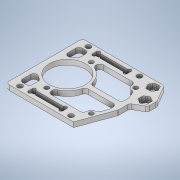
# Autodesk Inventor part: Trunk_vertical_frame_04
Saved by Autodesk Inventor 2020.4 (Build 244396000, 396)
## iProperties
Created: 2021-09-10
Part Number: Trunk_vertical_frame_04
Material: アルミニウム 2014-T4
Document SubType Name: Modeling
Designer: Masato Kubotera
Density: 2.8 g/cm^3
Appearance: 滑らか - 淡い灰色
Mass: 10.7602 g
Surface Area: 49.1447 cm^2
Volume: 3.84295 cm^3
Author: Masato Kubotera
Autodesk Inventor part; units mm, degrees
ref_plane "YZ Plane" through (0, 0, 0) normal (1, 0, 0) x (0, 1, 0)
ref_plane "XZ Plane" through (0, 0, 0) normal (0, 1, 0) x (-1, 0, 0)
ref_plane "XY Plane" through (0, 0, 0) normal (0, 0, 1) x (1, 0, 0)
derived "Trunk_vertical_frame_03.ipt"
sketch "スケッチ1" plane through (0, 0, 0) normal (0, 0, 1) x (1, 0, 0)
  circle A0 centre (0, 0) radius 11
  line L0 (1, 13.5) -> (28, 13.5) construction
  line L1 (28, 13.5) -> (28, -13.5) construction
  line L2 (28, -13.5) -> (1, -13.5) construction
  line L3 (1, -13.5) -> (1, 13.5) construction
  line L4 (1, 13.5) -> (28, -13.5) construction
  line L5 (28, 13.5) -> (1, -13.5) construction
  line L6 (-12, 16) -> (39.5, 16) construction
  line L7 (39.5, 16) -> (39.5, -16) construction
  line L8 (39.5, -16) -> (-12, -16) construction
  line L9 (-12, -16) -> (-12, 16) construction
  line L10 (-12, 16) -> (39.5, -16) construction
  line L11 (39.5, 16) -> (-12, -16) construction
  circle A1 centre (1, 13.5) radius 1.35
  arc A2 (0, 16) -> (-12, 10.583) centre (0, 0) ccw construction
  line L12 (-12, 0) -> (39.5, 0) construction
  circle A3 centre (28, 13.5) radius 1.35
  arc A4 (-12, -10.583) -> (0, -16) centre (0, 0) ccw construction
  circle A5 centre (28, -13.5) radius 1.35
  circle A6 centre (1, -13.5) radius 1.35
  arc A7 (0, 16.01) -> (-12.01, 10.5868) centre (0, 0) ccw construction
  line L13 (0, 16.01) -> (39.51, 16.01) construction
  line L14 (39.51, 16.01) -> (39.51, 13.26) construction
  line L15 (-12.01, 10.5868) -> (-12.01, 0) construction
  arc A8 (-11.4729, 11.1666) -> (-12.01, 9.8444) centre (-11.0278, 10.2156) ccw construction
  line L16 (-12.01, 10.5868) -> (-11.0278, 10.2156) construction
  arc A9 (39.51, 14.5251) -> (38.0251, 16.01) centre (38.7675, 15.2675) ccw construction
  line L17 (38.7675, 15.2675) -> (39.51, 16.01) construction
  arc A10 (38.0251, -16.01) -> (39.51, -14.5251) centre (38.7675, -15.2675) ccw construction
  line L18 (-12.01, -10.5868) -> (-12.01, 0) construction
  arc A11 (-12.01, -9.8444) -> (-11.4729, -11.1666) centre (-11.0278, -10.2156) ccw construction
  arc A12 (-12.01, -10.5868) -> (0, -16.01) centre (0, 0) ccw construction
  line L19 (0, -16.01) -> (39.51, -16.01) construction
  line L20 (39.51, 13.26) -> (42.01, 13.26) construction
  line L21 (42.01, 13.26) -> (42.01, -1.76) construction
  line L22 (42.01, -1.76) -> (39.51, -1.76) construction
  line L23 (39.51, -1.76) -> (39.51, -14.5251) construction
  line L24 (39.5, 13.25) -> (42, 13.25) construction
  line L25 (42, 13.25) -> (42, -1.75) construction
  line L26 (42, -1.75) -> (39.5, -1.75) construction
  line L27 (42, 5.75) -> (39.5, 5.75) construction
  arc A13 (42.01, 11.7751) -> (40.5251, 13.26) centre (41.2675, 12.5175) ccw construction
  line L28 (41.2675, 12.5175) -> (42.01, 13.26) construction
  arc A14 (40.5251, -1.76) -> (42.01, -0.2751) centre (41.2675, -1.0175) ccw construction
  circle A15 centre (-15.5, 19) radius 1.55 construction
  line L29 (-18, 22) -> (-13, 22) construction
  line L30 (-13, 22) -> (-13, -10.5) construction
  line L31 (-13, -10.5) -> (-18, -10.5) construction
  line L32 (-18, -10.5) -> (-18, 22) construction
  line L33 (-18, 22) -> (-13, -10.5) construction
  line L34 (-13, 22) -> (-18, -10.5) construction
  line L35 (-18, 5.75) -> (-13, 5.75) construction
  line L36 (-15.5, 22) -> (-15.5, -10.5) construction
  line L37 (-18, 13.25) -> (-15.5, 13.25) construction
  line L38 (-15.5, 13.25) -> (-15.5, -1.75) construction
  line L39 (-15.5, -1.75) -> (-18, -1.75) construction
  line L40 (-18, 13.25) -> (-15.5, -1.75) construction
  line L41 (-15.5, 13.25) -> (-18, -1.75) construction
  line L42 (-15.49, -1.76) -> (-18.01, -1.76) construction
  line L43 (-18.01, -1.76) -> (-18.01, 13.26) construction
  line L44 (-18.01, 13.26) -> (-15.49, 13.26) construction
  line L45 (-15.49, 13.26) -> (-15.49, -1.76) construction
  line L46 (-15.49, -1.76) -> (-18.01, 13.26) construction
  line L47 (-18.01, -1.76) -> (-15.49, 13.26) construction
  line L48 (-16.75, 13.26) -> (-16.75, -1.76) construction
  arc A16 (-18.01, 13.26) -> (-18.01, 11.16) centre (-18.01, 12.21) ccw construction
  arc A17 (-15.49, 11.16) -> (-15.49, 13.26) centre (-15.49, 12.21) ccw construction
  arc A18 (-18.01, 0.34) -> (-18.01, -1.76) centre (-18.01, -0.71) ccw construction
  arc A19 (-15.49, -1.76) -> (-15.49, 0.34) centre (-15.49, -0.71) ccw construction
  circle A20 centre (-15.5, -7.5) radius 1.55 construction
  line L49 (14.5, 16) -> (14.5, -16) construction
  circle A21 centre (42, 19) radius 1.55 construction
  line L50 (39.5, 22) -> (44.5, 22) construction
  line L51 (44.5, 22) -> (44.5, -10.5) construction
  line L52 (44.5, -10.5) -> (39.5, -10.5) construction
  line L53 (39.5, 22) -> (44.5, -10.5) construction
  line L54 (44.5, 22) -> (39.5, -10.5) construction
  line L55 (42, 22) -> (42, -10.5) construction
  circle A22 centre (42, -7.5) radius 1.55 construction
  line L56 (-12, -18.25) -> (27, -18.25) construction
  line L57 (27, -18.25) -> (27, -23.25) construction
  line L58 (27, -23.25) -> (-12, -23.25) construction
  line L59 (-12, -23.25) -> (-12, -18.25) construction
  line L60 (-12, -18.25) -> (27, -23.25) construction
  line L61 (27, -18.25) -> (-12, -23.25) construction
  line L62 (-3, -20.75) -> (18, -20.75) construction
  line L63 (18, -20.75) -> (18, -18.25) construction
  line L64 (-3, -18.25) -> (-3, -20.75) construction
  line L65 (-3, -20.75) -> (18, -18.25) construction
  line L66 (18, -20.75) -> (-3, -18.25) construction
  line L67 (-12, -20.75) -> (27, -20.75) construction
  line L68 (7.5, -18.25) -> (7.5, -23.25) construction
  line L69 (-3.01, -18.24) -> (18.01, -18.24)
  line L70 (18.01, -18.24) -> (18.01, -20.76)
  line L71 (18.01, -20.76) -> (-3.01, -20.76)
  line L72 (-3.01, -20.76) -> (-3.01, -18.24)
  line L73 (-3.01, -18.24) -> (18.01, -20.76) construction
  line L74 (18.01, -18.24) -> (-3.01, -20.76) construction
  circle A23 centre (-8, -20.75) radius 1.55
  circle A24 centre (23, -20.75) radius 1.55
  arc A25 (-0.91, -18.24) -> (-3.01, -18.24) centre (-1.96, -18.24) ccw
  arc A26 (18.01, -18.24) -> (15.91, -18.24) centre (16.96, -18.24) ccw
  line L75 (-3.01, -19.5) -> (18.01, -19.5) construction
  arc A27 (-3.01, -20.76) -> (-0.91, -20.76) centre (-1.96, -20.76) ccw
  arc A28 (15.91, -20.76) -> (18.01, -20.76) centre (16.96, -20.76) ccw
  circle A29 centre (-8, 20.75) radius 1.55
  line L76 (18.01, 20.76) -> (-3.01, 20.76)
  line L77 (-3.01, 19.5) -> (18.01, 19.5) construction
  line L78 (-3, 18.25) -> (-3, 20.75) construction
  line L79 (18, 20.75) -> (-3, 18.25) construction
  line L80 (-3, 20.75) -> (18, 18.25) construction
  line L81 (-3.01, 20.76) -> (-3.01, 18.24)
  line L82 (-3.01, 18.24) -> (18.01, 20.76) construction
  line L83 (-3.01, 18.24) -> (18.01, 18.24)
  arc A30 (-3.01, 18.24) -> (-0.91, 18.24) centre (-1.96, 18.24) ccw
  line L84 (18.01, 18.24) -> (-3.01, 20.76) construction
  line L85 (-12, 23.25) -> (-12, 18.25) construction
  arc A31 (-0.91, 20.76) -> (-3.01, 20.76) centre (-1.96, 20.76) ccw
  line L86 (7.5, 18.25) -> (7.5, 23.25) construction
  line L87 (-3, 20.75) -> (18, 20.75) construction
  line L88 (-12, 20.75) -> (27, 20.75) construction
  line L89 (27, 23.25) -> (-12, 23.25) construction
  line L90 (-12, 18.25) -> (27, 18.25) construction
  line L91 (-12, 18.25) -> (27, 23.25) construction
  line L92 (27, 18.25) -> (-12, 23.25) construction
  line L93 (27, 18.25) -> (27, 23.25) construction
  arc A32 (15.91, 18.24) -> (18.01, 18.24) centre (16.96, 18.24) ccw
  circle A33 centre (23, 20.75) radius 1.55
  line L94 (18, 20.75) -> (18, 18.25) construction
  line L95 (18.01, 18.24) -> (18.01, 20.76)
  arc A34 (18.01, 20.76) -> (15.91, 20.76) centre (16.96, 20.76) ccw
  line L96 (-18, 28.25) -> (44.5, 28.25) construction
  line L97 (-18, 28.25) -> (-23, 22) construction
  line L98 (44.5, 28.25) -> (47.5, 22) construction
  line L99 (-23, 22) -> (-23, -2.875) construction
  line L100 (47.5, 22) -> (47.5, -18.25) construction
  line L101 (47.5, -18.25) -> (37, -33.25) construction
  line L102 (-23, -2.875) -> (-33.5, -16) construction
  line L103 (-33.5, -16) -> (-33.5, -87) construction
  line L104 (37, -33.25) -> (37, -73.9) construction
  line L105 (37, -73.9) -> (23, -97) construction
  line L106 (23, -97) -> (-17, -97) construction
  line L107 (-17, -97) -> (-33.5, -87) construction
  circle A35 centre (-12, -92) radius 1.55 construction
  circle A36 centre (3, -92) radius 1.55 construction
  line L108 (-17, -97) -> (-17, -87) construction
  line L109 (-17, -87) -> (23, -87) construction
  line L110 (23, -87) -> (23, -97) construction
  line L111 (-17, -92) -> (23, -92) construction
  line L112 (3, -87) -> (3, -97) construction
  circle A37 centre (18, -92) radius 1.55 construction
  circle A38 centre (-13.5, -58.25) radius 1.55 construction
  line L113 (-23.5, -62.25) -> (27, -62.25) construction
  line L114 (27, -62.25) -> (27, -77) construction
  line L115 (27, -77) -> (-23.5, -77) construction
  line L116 (-23.5, -77) -> (-23.5, -62.25) construction
  line L117 (-23.5, -33.25) -> (27, -33.25) construction
  line L118 (27, -33.25) -> (27, -54.25) construction
  line L119 (27, -54.25) -> (-23.5, -54.25) construction
  line L120 (-23.5, -54.25) -> (-23.5, -33.25) construction
  circle A39 centre (-13.5, -58.25) radius 4 construction
  line L121 (-14, 23.25) -> (27, 23.25)
  line L122 (27, 23.25) -> (34.2657, 3.3202)
  line L123 (34.2657, 3.3202) -> (34.2657, -3.3202)
  line L124 (-14, -23.25) -> (27, -23.25)
  line L125 (27, -23.25) -> (34.2657, -3.3202)
  circle A40 centre (33, 19) radius 2.25
  line L126 (34.5935, 16.24) -> (31.4065, 16.24)
  line L127 (31.4065, 16.24) -> (29.813, 19)
  line L128 (29.813, 19) -> (31.4065, 21.76)
  line L129 (31.4065, 21.76) -> (34.5935, 21.76)
  line L130 (34.5935, 21.76) -> (36.187, 19)
  line L131 (36.187, 19) -> (34.5935, 16.24)
  circle A41 centre (37.2262, 9.9369) radius 2.25
  line L132 (37.2262, 6.7499) -> (34.4662, 8.3434)
  line L133 (34.4662, 8.3434) -> (34.4662, 11.5304)
  line L134 (34.4662, 11.5304) -> (37.2262, 13.1239)
  line L135 (37.2262, 13.1239) -> (39.9862, 11.5304)
  line L136 (39.9862, 11.5304) -> (39.9862, 8.3434)
  line L137 (39.9862, 8.3434) -> (37.2262, 6.7499)
  line L138 (33, 19) -> (37.2262, 9.9369) construction
  line L139 (27, 23.25) -> (35.4537, 23.25)
  line L140 (35.4537, 23.25) -> (41.4762, 12.8188)
  line L141 (41.4762, 12.8188) -> (41.4762, 7.4832)
  line L142 (41.4762, 7.4832) -> (34.2657, 3.3202)
  circle A42 centre (28, 13.5) radius 2.4 construction
  arc A43 (32.4565, 21.76) -> (30.8815, 20.8507) centre (31.9315, 20.8507) ccw
  arc A44 (30.338, 19.9093) -> (30.338, 18.0907) centre (30.863, 19) ccw
  arc A45 (30.8815, 17.1493) -> (32.4565, 16.24) centre (31.9315, 17.1493) ccw
  arc A46 (33.5435, 16.24) -> (35.1185, 17.1493) centre (34.0685, 17.1493) ccw
  arc A47 (35.662, 18.0907) -> (35.662, 19.9093) centre (35.137, 19) ccw
  arc A48 (35.1185, 20.8507) -> (33.5435, 21.76) centre (34.0685, 20.8507) ccw
  arc A49 (38.1355, 12.5989) -> (36.3169, 12.5989) centre (37.2262, 12.0739) ccw
  arc A50 (35.3755, 12.0554) -> (34.4662, 10.4804) centre (35.3755, 11.0054) ccw
  arc A51 (34.4662, 9.3934) -> (35.3755, 7.8184) centre (35.3755, 8.8684) ccw
  arc A52 (36.3169, 7.2749) -> (38.1355, 7.2749) centre (37.2262, 7.7999) ccw
  arc A53 (39.0769, 7.8184) -> (39.9862, 9.3934) centre (39.0769, 8.8684) ccw
  arc A54 (39.9862, 10.4804) -> (39.0769, 12.0554) centre (39.0769, 11.0054) ccw
  arc A55 (-9.1456, 18.25) -> (-6.8544, 18.25) centre (-8, 20.75) ccw
  line L143 (-6.8544, 18.25) -> (-5, 18.25)
  line L144 (-5, 18.25) -> (-5, 11.4564)
  line L145 (4, 15.75) -> (4, 11.8427)
  line L146 (4, 15.75) -> (26.9103, 15.75)
  arc A56 (26.9103, 15.75) -> (28, 11) centre (28, 13.5) ccw
  line L147 (28, 11) -> (29.3372, 11)
  line L148 (31.2657, 5.71) -> (31.2657, 1.5)
  line L149 (29.3372, 11) -> (31.2657, 5.71)
  arc A57 (-5, 11.4564) -> (-11, 5.9372) centre (0, 0) ccw
  arc A58 (12.4097, 1.5) -> (4, 11.8427) centre (0, 0) ccw
  line L150 (4, -15.75) -> (4, -11.8427)
  line L151 (4, -15.75) -> (26.9103, -15.75)
  arc A59 (28, -11) -> (26.9103, -15.75) centre (28, -13.5) ccw
  line L152 (31.2657, -5.71) -> (31.2657, -1.5)
  line L153 (29.3372, -11) -> (31.2657, -5.71)
  arc A60 (4, -11.8427) -> (12.4097, -1.5) centre (0, 0) ccw
  line L154 (28, -11) -> (29.3372, -11)
  arc A61 (-11.4565, -94.76) -> (-9.8815, -93.8507) centre (-10.9315, -93.8507) ccw construction
  line L155 (-9.338, -92.9093) -> (-9.8815, -93.8507) construction
  arc A62 (-9.338, -92.9093) -> (-9.338, -91.0907) centre (-9.863, -92) ccw construction
  line L156 (-9.8815, -90.1493) -> (-9.338, -91.0907) construction
  arc A63 (-9.8815, -90.1493) -> (-11.4565, -89.24) centre (-10.9315, -90.1493) ccw construction
  line L157 (-12.5435, -89.24) -> (-11.4565, -89.24) construction
  arc A64 (-12.5435, -89.24) -> (-14.1185, -90.1493) centre (-13.0685, -90.1493) ccw construction
  line L158 (-14.662, -91.0907) -> (-14.1185, -90.1493) construction
  arc A65 (-14.662, -91.0907) -> (-14.662, -92.9093) centre (-14.137, -92) ccw construction
  line L159 (-14.1185, -93.8507) -> (-14.662, -92.9093) construction
  arc A66 (-14.1185, -93.8507) -> (-12.5435, -94.76) centre (-13.0685, -93.8507) ccw construction
  line L160 (-11.4565, -94.76) -> (-12.5435, -94.76) construction
  arc A67 (5.662, -92.9093) -> (5.662, -91.0907) centre (5.137, -92) ccw construction
  line L161 (5.1185, -90.1493) -> (5.662, -91.0907) construction
  line L162 (5.662, -92.9093) -> (5.1185, -93.8507) construction
  arc A68 (3.5435, -94.76) -> (5.1185, -93.8507) centre (4.0685, -93.8507) ccw construction
  arc A69 (5.1185, -90.1493) -> (3.5435, -89.24) centre (4.0685, -90.1493) ccw construction
  line L163 (2.4565, -89.24) -> (3.5435, -89.24) construction
  arc A70 (2.4565, -89.24) -> (0.8815, -90.1493) centre (1.9315, -90.1493) ccw construction
  line L164 (0.338, -91.0907) -> (0.8815, -90.1493) construction
  arc A71 (0.338, -91.0907) -> (0.338, -92.9093) centre (0.863, -92) ccw construction
  line L165 (0.8815, -93.8507) -> (0.338, -92.9093) construction
  arc A72 (0.8815, -93.8507) -> (2.4565, -94.76) centre (1.9315, -93.8507) ccw construction
  line L166 (3.5435, -94.76) -> (2.4565, -94.76) construction
  arc A73 (20.662, -92.9093) -> (20.662, -91.0907) centre (20.137, -92) ccw construction
  line L167 (20.1185, -90.1493) -> (20.662, -91.0907) construction
  line L168 (20.662, -92.9093) -> (20.1185, -93.8507) construction
  arc A74 (18.5435, -94.76) -> (20.1185, -93.8507) centre (19.0685, -93.8507) ccw construction
  arc A75 (20.1185, -90.1493) -> (18.5435, -89.24) centre (19.0685, -90.1493) ccw construction
  line L169 (17.4565, -89.24) -> (18.5435, -89.24) construction
  arc A76 (17.4565, -89.24) -> (15.8815, -90.1493) centre (16.9315, -90.1493) ccw construction
  line L170 (15.338, -91.0907) -> (15.8815, -90.1493) construction
  arc A77 (15.338, -91.0907) -> (15.338, -92.9093) centre (15.863, -92) ccw construction
  line L171 (15.8815, -93.8507) -> (15.338, -92.9093) construction
  arc A78 (15.8815, -93.8507) -> (17.4565, -94.76) centre (16.9315, -93.8507) ccw construction
  line L172 (18.5435, -94.76) -> (17.4565, -94.76) construction
  line L173 (12.4097, 1.5) -> (31.2657, 1.5)
  line L174 (31.2657, -1.5) -> (12.4097, -1.5)
  line L175 (-14, 23.25) -> (-14, -23.25)
  line L176 (-6.8544, -18.25) -> (-5, -18.25)
  line L177 (-5, -18.25) -> (-5, -11.4564)
  arc A79 (-11, -5.9372) -> (-5, -11.4564) centre (0, 0) ccw
  line L178 (-9.1456, 18.25) -> (-11, 18.25)
  line L179 (-11, 18.25) -> (-11, 5.9372)
  arc A80 (-6.8544, -18.25) -> (-9.1456, -18.25) centre (-8, -20.75) ccw
  line L180 (-11, -18.25) -> (-11, -5.9372)
  line L181 (-9.1456, -18.25) -> (-11, -18.25)
  point P0 (14.5, 0)
  point P1 (-15.5, 5.75)
  point P2 (-16.75, 5.75)
  point P3 (14.5, 0)
  point P4 (42, 5.75)
  point P5 (42, 5.75)
  point P6 (7.5, -20.75)
  point P7 (7.5, -19.5)
  point P8 (7.5, -19.5)
  point P9 (7.5, -19.5)
  point P10 (7.5, -19.5)
  point P11 (7.5, 20.75)
  point P12 (7.5, 19.5)
  point P13 (7.5, 19.5)
  point P14 (7.5, 19.5)
  point P15 (7.5, 19.5)
  point P16 (29.813, 19)
  point P17 (36.187, 19)
  point P18 (34.5935, 21.76)
  point P19 (34.4662, 11.5304)
  point P20 (34.4662, 8.3434)
  point P21 (37.2262, 6.7499)
  point P22 (39.9862, 8.3434)
  point P23 (39.9862, 11.5304)
  point P24 (35.1185, 20.8507)
  point P25 (35.662, 19.9093)
  point P26 (35.662, 18.0907)
  point P27 (35.1185, 17.1493)
  point P28 (33.5435, 16.24)
  point P29 (32.4565, 16.24)
  point P30 (30.8815, 17.1493)
  point P31 (30.338, 18.0907)
  point P32 (30.338, 19.9093)
  point P33 (33.5435, 21.76)
  point P34 (15.91, 18.24)
  point P35 (-0.91, 20.76)
  point P36 (15.91, 20.76)
  point P37 (38.1326, 16.1038)
  point P38 (39.8174, 15.2498)
  point P39 (39.9862, 10.4804)
  point P40 (39.9862, 9.3934)
  point P41 (39.0769, 7.8184)
  point P42 (38.1355, 7.2749)
  point P43 (36.3169, 7.2749)
  point P44 (35.3755, 7.8184)
  point P45 (34.4662, 9.3934)
  point P46 (34.4662, 10.4804)
  point P47 (35.3755, 12.0554)
  point P48 (15.91, -20.76)
  point P49 (-0.91, -20.76)
  point P50 (15.91, -18.24)
  point P51 (41.4762, 13.26)
  point P52 (41.4762, 13.5466)
  point P53 (39.0769, 12.0554)
  point P54 (3, -89.25)
  point P55 (-10.4065, -94.76)
  point P56 (-8.813, -92)
  point P57 (-10.4065, -89.24)
  point P58 (-13.5935, -89.24)
  point P59 (-13.5935, -89.24)
  point P60 (-15.187, -92)
  point P61 (-13.5935, -94.76)
  point P62 (-15.187, -92)
  point P63 (-8.813, -92)
  point P64 (3, -92)
  point P65 (6.187, -92)
  point P66 (6.187, -92)
  point P67 (4.5935, -89.24)
  point P68 (4.5935, -94.76)
  point P69 (3, -92)
  point P70 (3, -92)
  point P71 (1.4065, -89.24)
  point P72 (1.4065, -89.24)
  point P73 (-0.187, -92)
  point P74 (-0.187, -92)
  point P75 (1.4065, -94.76)
  point P76 (18, -92)
  point P77 (21.187, -92)
  point P78 (21.187, -92)
  point P79 (19.5935, -89.24)
  point P80 (19.5935, -94.76)
  point P81 (18, -92)
  point P82 (18, -92)
  point P83 (16.4065, -89.24)
  point P84 (16.4065, -89.24)
  point P85 (14.813, -92)
  point P86 (14.813, -92)
  point P87 (16.4065, -94.76)
  point P88 (41.0563, 13.5461)
  point P89 (41.2215, 13.26)
  dimension "d11" = 4.5
  dimension "d12" = 10
  dimension "d13" = 5.52
  dimension "d14" = 4.25
  dimension "d15" = 4.5
  dimension "d16" = 5.52
  dimension "d17" = 115
  dimension "d18" = 10
  dimension "d20" = 4.25
  dimension "d21" = 4.8
  dimension "d22" = 4.25
  dimension "d23" = 1.05
  dimension "d26" = 360
  dimension "d28" = 1.05
  dimension "d31" = 360
  dimension "d37" = 2.75
  dimension "d38" = 2
  dimension "d39" = 3
  dimension "d40" = 2.5
  dimension "d41" = 2.5
  dimension "d43" = 3
  dimension "d44" = 2
  dimension "d45" = 1.5
  dimension "d52" = 0
  dimension "d53" = 3
  dimension "d57" = 4.25
  dimension "d58" = 3
  dimension "d59" = 3
  measures "d11" diameter of A40
  measures "d12" horizontal distance of A40.centre A33.centre
  measures "d13" distance of L126.start L129.end
  measures "d14" vertical distance of A40.centre L121.end
  measures "d15" diameter of A41
  measures "d16" distance between parallel lines of L132 L135
  measures "d17" angle of L121 L138
  measures "d18" distance of L138.start L138.end
  measures "d20" horizontal distance of L141.end A41.centre
  measures "d21" diameter of A42
  measures "d22" distance from line of L138.start L140
  measures "d23" radius of A43
  measures "d28" radius of A49
  measures "d37" radius of A55
  measures "d38" distance from line of L78.start L144
  measures "d39" distance from line of L145 L0.start
  measures "d40" distance from line of L145.start L90
  measures "d41" radius of A56
  measures "d43" distance between parallel lines of L123 L148
  measures "d44" distance between parallel lines of L122 L149
  measures "d45" radial gap between concentric circles of A0 A57
  measures "d52" vertical distance of L89.end L121.start
  measures "d53" distance of L152.end L148.end
  measures "d57" distance from line of L142 A41.centre
  measures "d58" distance edge to line of A0 L175
  measures "d59" distance from line of L121.start L179
extrude "押し出し1" add sketch "スケッチ1" along normal blind 3 contours L121 L122 L123 L125 L124 L175 | L139 L140 L141 L142 L122
extrude "押し出し2" add sketch "スケッチ1" along normal blind 0.8 contours A46 L126 | L126 L127 L128 L129 L130 L131 | L131 A46 | A45 L126 | L131 A47 | A45 L127 | L130 A47 | A44 L127 | L130 A48 | A44 L128 | L129 A48 | A43 L128 | L129 A43 | A52 L132 | L132 L133 L134 L135 L136 L137 | L137 A52 | A51 L132 | L137 A53 | A51 L133 | L136 A53 | A50 L133 | L136 A54 | A50 L134 | L135 A54 | A49 L134 | L135 A49
fillet "フィレット1" radius 2 26 edges at (-5, 18.25, 1.5) (-5, 11.4564, 1.5) (4, 11.8427, 1.5) (4, 15.75, 1.5) (4, -15.75, 1.5) (4, -11.8427, 1.5) (31.2657, -5.71, 1.5) (29.3372, -11, 1.5) (26.9103, -15.75, 1.5) (26.9103, 15.75, 1.5) (29.3372, 11, 1.5) (31.2657, 5.71, 1.5) (-5, -11.4564, 1.5) (-5, -18.25, 1.5) (12.4097, 1.5, 1.5) (12.4097, -1.5, 1.5) (31.2657, 1.5, 1.5) (31.2657, -1.5, 1.5) (-11, 18.25, 1.5) (-9.1456, 18.25, 1.5) (-6.8544, 18.25, 1.5) (-11, 5.9372, 1.5) (-11, -5.9372, 1.5) (-11, -18.25, 1.5) (-9.1456, -18.25, 1.5) (-6.8544, -18.25, 1.5)
fillet "フィレット2" radius 2 7 edges at (35.4537, 23.25, 1.5) (41.4762, 12.8188, 1.5) (41.4762, 7.4832, 1.5) (34.2657, 3.3202, 1.5) (34.2657, -3.3202, 1.5) (-14, -23.25, 1.5) (-14, 23.25, 1.5)
equation "\"d15\" = d11"
equation "\"d16\" = d13"
equation "\"d20\" = d14"
equation "\"d22\" = d14"
equation "\"d28\" = d23"
equation "\"d38\" = d33"
equation "\"d40\" = d8"
equation "\"d41\" = d9"
equation "\"d9\" = d8"
equation "\"d33\" = 2"
equation "\"d8\" = 2.5"
